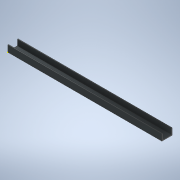
# Autodesk Inventor part: alCchannel
Saved by Autodesk Inventor 2020 (Build 240168000, 168)
## iProperties
Created: 2020-03-02
Part Number: alCchannel
Material: Generic
Document SubType Name: Modeling
Designer: akend
Density: 1 g/cm^3
Appearance: Gray
Author: akend
Autodesk Inventor part; units mm, degrees
ref_plane "YZ Plane" through (0, 0, 0) normal (1, 0, 0) x (0, 1, 0)
ref_plane "XZ Plane" through (0, 0, 0) normal (0, 1, 0) x (-1, 0, 0)
ref_plane "XY Plane" through (0, 0, 0) normal (0, 0, 1) x (1, 0, 0)
sketch "Sketch1" plane through (0, 0, 0) normal (1, 0, 0) x (0, 1, 0)
  point P0 (0, 0)
sketch "Sketch2" plane through (0, 0, 0) normal (1, 0, 0) x (0, 1, 0)
  line L0 (0, 0) -> (0, -22.5)
  line L1 (0, 0) -> (14, 0)
  line L2 (0, -22.5) -> (14, -22.5)
  line L3 (14, 0) -> (14, -1.588)
  line L4 (14, -1.588) -> (1.588, -1.588)
  line L5 (1.588, -1.588) -> (1.588, -20.912)
  line L6 (1.588, -20.912) -> (14, -20.912)
  line L7 (14, -20.912) -> (14, -22.5)
  dimension "d0" = 22.5
  dimension "d1" = 14
  dimension "d2" = 14
  dimension "d3" = 1.588
  dimension "d4" = 12.412
  dimension "d5" = 19.324
  constraints: 16 end point, 3 perpendicular, 2 horizontal, 2 vertical, 1 point on line
  measures "d0" distance of L0.start L0.end
  measures "d1" distance of L0.start L1.end
  measures "d2" distance of L0.end L2.end
  measures "d3" distance of L1.end L3.end
  measures "d4" distance of L3.end L4.end
  measures "d5" distance of L4.end L5.end
extrude "Extrusion1" add sketch "Sketch2" along normal blind 334.01
body "Solid1"
